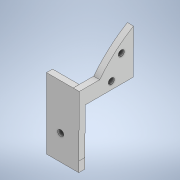
# Autodesk Inventor part: encoderholderL
Saved by Autodesk Inventor 2022 (Build 260153000, 153)
## iProperties
Created: 2025-02-10
Part Number: encoderholderL
Material: Типовые
Document SubType Name: Modeling
Designer: korsh624
Density: 1 g/cm^3
Appearance: По умолчанию
Author: korsh624
Autodesk Inventor part; units mm, degrees
ref_plane "YZ Plane" through (0, 0, 0) normal (1, 0, 0) x (0, 1, 0)
ref_plane "XZ Plane" through (0, 0, 0) normal (0, 1, 0) x (-1, 0, 0)
ref_plane "XY Plane" through (0, 0, 0) normal (0, 0, 1) x (1, 0, 0)
sketch "Эскиз1" plane through (0, 0, 0) normal (0, 0, 1) x (1, 0, 0)
  circle A0 centre (-3.8814, -5.2176) radius 1.5 projected
  line L0 (-10.8201, 1.8432) -> (-11.0949, -29.6556) projected
  line L1 (4.4719, -79.3628) -> (5.5191, 40.6326) projected
  line L2 (-9.8587, -12.7657) -> (-5.4656, -12.804) projected
  line L3 (-10.9475, -12.7562) -> (5.315, -12.7562)
  line L4 (5.315, -12.7562) -> (5.315, 17.2438)
  line L5 (5.315, 17.2438) -> (-10.9475, 17.2438)
  line L6 (-10.9475, 17.2438) -> (-10.9475, -12.7562)
  point P0 (0, 0)
  point P1 (5.1784, 1.5986)
  point P2 (5.0531, -12.7562)
  dimension "d0" = 30
  constraints: 8 end point, 2 parallel, 2 point on line, 1 horizontal, 1 perpendicular, 1 other
  measures "d0" distance of L4.end L3.end
extrude "Выдавливание1" add sketch "Эскиз1" along normal blind 3 contours L3 L6 L5 L1
sketch "Эскиз2" plane through (5.315, 17.2438, 3) normal (1, -0.0087, 0) x (0, 0, -1)
  spline S0 degree 3 poles (-15.9024, -5.0587) (-16.7308, -5.0587) (-17.4024, -4.3871) (-17.4024, -3.5587) (-17.4024, -2.7303) (-16.7308, -2.0587) (-15.9024, -2.0587) (-15.074, -2.0587) (-14.4024, -2.7303) (-14.4024, -3.5587) (-14.4024, -4.3871) (-15.074, -5.0587) (-15.9024, -5.0587) knots 0 0 0 0 0.25 0.25 0.25 0.5 0.5 0.5 0.75 0.75 0.75 1 1 1 1 projected
  spline S1 degree 3 poles (-20.7708, 4.5722) (-21.5992, 4.5722) (-22.2708, 5.2438) (-22.2708, 6.0722) (-22.2708, 6.9006) (-21.5992, 7.5722) (-20.7708, 7.5722) (-19.9424, 7.5722) (-19.2708, 6.9006) (-19.2708, 6.0722) (-19.2708, 5.2438) (-19.9424, 4.5722) (-20.7708, 4.5722) knots 0 0 0 0 0.25 0.25 0.25 0.5 0.5 0.5 0.75 0.75 0.75 1 1 1 1 projected
  line L0 (0, -30.0011) -> (0, 0) projected
  line L1 (0, -7.2902) -> (-26.751, -7.2902)
  spline S2 degree 3 poles (-117.3896, -42.4533) (-114.4523, -72.8485) (-88.8364, -96.6103) (-57.6706, -96.6103) (-24.5335, -96.6103) (2.3293, -69.7475) (2.3293, -36.6104) (2.3293, -3.4733) (-24.5335, 23.3896) (-57.6706, 23.3896) (-89.3782, 23.3896) (-115.3412, -1.2057) (-117.5222, -32.3587) knots 0 0 0 0 0.2 0.2 0.2 0.4 0.4 0.4 0.6 0.6 0.6 0.8 0.8 0.8 0.8 projected
  line L2 (-26.751, -7.2902) -> (-26.751, 14.8198)
  line L3 (-10.1308, 0) -> (0, 0)
  point P0 (3, -17.2895)
  point P1 (-15.9024, -5.0587)
  point P2 (-20.7708, 4.5722)
  constraints: 6 end point, 1 horizontal, 1 perpendicular, 1 point on line, 1 vertical, 2 other
extrude "Выдавливание2" add sketch "Эскиз2" against normal blind 3 contours L1 S2 L3 L0 | L1 L2 S2
sketch "Эскиз3" plane through (0, 0, 0) normal (0, 0, -1) x (-1, 0, 0)
  line L0 (-5.315, 17.2438) -> (10.9475, 17.2438) projected
  line L1 (10.9475, -12.7562) -> (-5.0531, -12.7562) projected
  line L2 (10.9475, 17.2438) -> (10.9475, -12.7562) projected
  line L3 (-5.315, 17.2438) -> (10.9475, 17.2438) projected
  line L4 (-5.0531, -12.7562) -> (-5.315, 17.2438) projected
  circle A0 centre (3.8814, -5.2176) radius 1.5 projected
  point P0 (0, 0)
extrude "Выдавливание3" add sketch "Эскиз3" against normal blind 6
sketch "Эскиз4" plane through (0, 0, 0) normal (0, 0, -1) x (-1, 0, 0)
  line L0 (10.9475, -12.7562) -> (-5.0531, -12.7562) projected
  line L1 (10.9475, 17.2438) -> (10.9475, -12.7562) projected
  line L2 (-5.315, 17.2438) -> (10.9475, 17.2438) projected
  line L3 (-5.0531, -12.7562) -> (-5.315, 17.2438) projected
  circle A0 centre (3.8814, -5.2176) radius 1.5 projected
  point P0 (0, 0)
extrude "Выдавливание4" cut sketch "Эскиз4" against normal blind 3
sketch "Эскиз5" plane through (-10.9475, -12.7562, 3) normal (0, -1, 0) x (1, 0, 0)
  line L0 (0, 0) -> (16.0006, 0) projected
  line L1 (16.0006, 0) -> (16.0006, 3) projected
  line L2 (0, 3) -> (16.0006, 3) projected
  line L3 (0, 0) -> (0, 3) projected
  point P0 (10.9475, -3)
extrude "Выдавливание5" add sketch "Эскиз5" along normal blind 5
mirror "Зеркальное отражение1" about plane through (5.2513, 9.9539, 29.751) normal (0, 0, 1) of "Выдавливание3", "Выдавливание2", "Выдавливание5"
sketch "Эскиз7" plane through (5.315, 17.2438, 13.1308) normal (1, -0.0087, 0) x (0, 0, -1)
  ellipse E0 centre (-44.6759, -33.7501) end of major axis (-85.7491, 7.3732) minor radius 55.9525 (0, 0) -> (-16.6202, 14.8198) ccw projected
  line L0 (0, 0) -> (0, -43.3652)
  line L1 (-16.6202, 18.912) -> (20.2447, 18.912)
  line L2 (20.2447, 18.912) -> (20.2447, -40.2119)
  line L3 (20.2447, -40.2119) -> (-16.6202, -40.2119)
  line L4 (-16.6202, -40.2119) -> (-16.6202, 18.912)
  line L5 (-46.3712, -30.1408) -> (-43.3712, -30.1408) projected
  line L6 (-43.3712, -30.1408) -> (-60.2207, -30.1408)
  line L7 (-60.2207, -30.1408) -> (-60.2207, 23.0222)
  line L8 (-60.2207, 23.0222) -> (-43.3712, 23.0222)
  line L9 (-43.3712, 23.0222) -> (-43.3712, -30.1408)
  point P0 (13.1308, -17.2895)
  constraints: 18 end point, 4 parallel, 2 horizontal, 2 perpendicular, 1 vertical, 1 other
extrude "Выдавливание6" cut sketch "Эскиз7" against normal blind 30
sketch "Эскиз8" plane through (5.0531, -17.7562, 6) normal (1, 0, 0) x (0, 0, -1)
  line L0 (3, 5) -> (0, 5) projected
  line L1 (0, 5) -> (0, 0) projected
  line L2 (3, 0) -> (0, 0) projected
  line L3 (3, 5) -> (3, 0) projected
  point P0 (6, 17.7562)
extrude "Выдавливание7" cut sketch "Эскиз8" against normal blind 30
